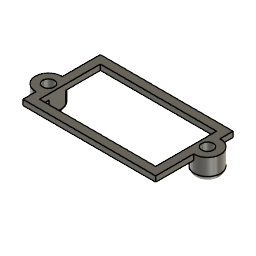
ServoMount_v1 (Autodesk Fusion 360 design; units mm, degrees)
Autodesk Fusion 360 part; units mm, degrees
sketch "Sketch1" plane through (0, 0, 0) normal (0, 0, 1) x (1, 0, 0)
  line L0 (-24.24, -4.5) -> (-24.24, -2) construction
  line L1 (24.24, -7) -> (21, -7) construction
  line L2 (-24.24, 2) -> (-21, 2)
  line L3 (-24.24, -4.5) -> (-24.24, -7) construction
  circle A0 centre (-24.24, 4.5) radius 2.5 construction
  line L4 (-24.24, -2) -> (-21, -2) construction
  line L5 (24.24, 7) -> (21, 7) construction
  line L6 (21, -11) -> (-21, 11) construction
  circle A1 centre (-24.24, -4.5) radius 2.5 construction
  line L7 (-21, -11) -> (-21, 11)
  line L8 (24.24, 2) -> (21, 2) construction
  line L9 (-24.24, 0) -> (24.24, 0) construction
  line L10 (24.24, 4.5) -> (24.24, -4.5) construction
  line L11 (-24.24, -7) -> (-21, -7)
  line L12 (-21, 11) -> (21, 11)
  line L13 (-21, -11) -> (21, 11) construction
  line L14 (-24.24, 4.5) -> (-24.24, -4.5) construction
  line L15 (-24.24, 4.5) -> (-24.24, 2) construction
  line L16 (-24.24, 4.5) -> (-24.24, 7) construction
  line L17 (-24.24, 7) -> (-21, 7) construction
  circle A2 centre (24.24, -4.5) radius 2.5 construction
  line L18 (21, 11) -> (21, -11)
  line L19 (24.24, -2) -> (21, -2) construction
  line L20 (24.24, 4.5) -> (24.24, 7) construction
  line L21 (21, -11) -> (-21, -11)
  circle A3 centre (24.24, 4.5) radius 2.5 construction
  circle A4 centre (24.24, 4.5) radius 2.1
  circle A5 centre (-24.24, -4.5) radius 2.1
  line L22 (-24, 14) -> (24, 14)
  line L23 (24, 14) -> (24, -14)
  line L24 (24, -14) -> (-24, -14)
  line L25 (-24, -14) -> (-24, 14)
  line L26 (-24, 14) -> (24, -14) construction
  line L27 (24, 14) -> (-24, -14) construction
  circle A6 centre (-24.24, -4.5) radius 4.76
  circle A7 centre (24.24, 4.5) radius 4.76
  dimension "d1" = 42
  dimension "d2" = 22
  dimension "d3" = 48.48
  dimension "d4" = 9
  dimension "d5" = 9
  dimension "d6" = 5
  dimension "d7" = 5
  dimension "d8" = 5
  dimension "d9" = 5
  dimension "d10" = 4.2
  dimension "d11" = 4.2
  dimension "d12" = 3
  dimension "d13" = 3
  constraint horizontal L21
  constraint perpendicular L7 L21
  constraint parallel L12 L21
  constraint parallel L7 L18
  constraint coincident origin L6
  constraint coincident origin L13
  constraint midpoint origin L9
  constraint perpendicular L9 L18
  constraint midpoint L9.end L10
  constraint midpoint L9.start L14
  constraint coincident L10.start L20.start
  constraint coincident L10.end A2.centre
  constraint coincident A0.centre L14.start
  constraint coincident L0.start L3.start
  constraint coincident L16.end A0
  constraint vertical L16
  constraint coincident L17.end L7
  constraint perpendicular L7 L17
  constraint coincident L2.start A0
  constraint coincident L2.start L14
  constraint coincident L2.end L7
  constraint perpendicular L2 L7
  constraint coincident L0.end A1
  constraint coincident L0.end L14
  constraint coincident L3.end A1
  constraint parallel L3 L14
  constraint coincident L4.end L7
  constraint perpendicular L4 L7
  constraint coincident L11.end L7
  constraint perpendicular L7 L11
  constraint coincident L5.start A3
  constraint parallel L10 L20
  constraint coincident L5.end L18
  constraint perpendicular L5 L18
  constraint coincident L8.start L10
  constraint coincident L8.start A3
  constraint coincident L8.end L18
  constraint tangent L8 A3
  constraint coincident L19.start A2
  constraint coincident L19.start L10
  constraint coincident L19.end L18
  constraint tangent A2 L19
  constraint coincident L1.start A2
  constraint coincident L1.end L18
  constraint tangent L1 A2
  constraint perpendicular L1 L18
  constraint concentric A3 A4
  constraint concentric A1 A5
  constraint horizontal L22
  constraint perpendicular L22 L23
  constraint parallel L22 L24
  constraint parallel L23 L25
  constraint coincident L26 origin
  constraint coincident L27 origin
  constraint concentric A1 A6
  constraint concentric A3 A7
  measures "d1" distance of L12.end L6.end
  measures "d2" distance of L7.start L6.end
  measures "d3" distance of L9.start L9.end
  measures "d4" distance of L10.start L10.end
  measures "d5" distance of L0.start A0.centre
  measures "d6" diameter of A3
  measures "d7" diameter of A2
  measures "d8" diameter of A0
  measures "d9" diameter of A1
  measures "d10" diameter of A4
  measures "d11" diameter of A5
  measures "d12" distance of L12 L22
  measures "d13" distance of L18 L23
extrude "Extrude1" add sketch "Sketch1" along normal blind 2 contours L2 L7 L12 L18 L22 L23 L25 A7 | L2 L7 L25 A6 | L7 L11 A5 L25 A6 | A5 L25 A6 | L7 L18 L21 L23 L24 L25 A6 A7 | L7 L11 L25 A6 | A4 L23 A7 | L18 A4 L23 A7
extrude "Extrude2" add sketch "Sketch1" against normal blind 4 contours L7 L11 A5 L25 A6 | A5 L25 A6 | L7 L11 L25 A6 | A4 L23 A7 | L18 A4 L23 A7
extrude "Extrude3" add sketch "Sketch1" against normal blind 2 from surface at -4 contours L7 L11 A5 L25 A6 | A5 L25 A6 | A5 L25 | A5 L25 | L7 L11 L25 A6 | A4 L23 A7 | L18 A4 L23 A7 | A4 L23 | A4 L23
fillet "Fillet1" radius 2 2 edges at (-29, -4.5, -6) (29, 4.5, -6)
fillet "Fillet2" radius 1 3 edges at (21, 1.0129, -2) (21, 4.5, -5.9415) (21, 7.9871, -2)
fillet "Fillet3" radius 1 3 edges at (-21, -7.9871, -2) (-21, -4.5, -5.9415) (-21, -1.0129, -2)
